Autodesk Fusion 360 part; units mm, degrees
(part 6 of 40)
  line L2344 (251.8229, 91.113) -> (251.9751, 91.0416) construction
  line L2345 (251.9751, 91.0416) -> (252.0973, 90.9849) construction
  line L2346 (252.0973, 90.9849) -> (252.1892, 90.9427) construction
  line L2347 (252.1892, 90.9427) -> (252.2505, 90.9147) construction
  line L2348 (252.2505, 90.9147) -> (252.2812, 90.9007) construction
  spline S31 degree 5 poles (243.2435, 97.4897) (243.2592, 97.4632) (243.2914, 97.4105) (243.3417, 97.3328) (243.4127, 97.2319) (243.5068, 97.1094) (243.6047, 96.9894) (243.7049, 96.8711) (243.8064, 96.7536) (243.9087, 96.6366) (244.012, 96.5203) (244.1164, 96.4049) (244.2223, 96.2906) (244.3301, 96.1776) (244.4397, 96.066) (244.551, 95.9556) (244.6636, 95.8463) (244.7775, 95.7378) (244.8923, 95.6302) (245.008, 95.5233) (245.1247, 95.4172) (245.2425, 95.3119) (245.3612, 95.2074) (245.4811, 95.1039) (245.602, 95.0012) (245.7239, 94.8993) (245.8468, 94.7983) (245.9706, 94.698) (246.0953, 94.5985) (246.2208, 94.4997) (246.3471, 94.4016) (246.4743, 94.3043) (246.6023, 94.2077) (246.7311, 94.1119) (246.8608, 94.0168) (246.9912, 93.9224) (247.1225, 93.8288) (247.2544, 93.7358) (247.3872, 93.6436) (247.5206, 93.552) (247.6548, 93.4612) (247.7897, 93.371) (247.9253, 93.2815) (248.0615, 93.1927) (248.1985, 93.1045) (248.3362, 93.0171) (248.4745, 92.9303) (248.6135, 92.8442) (248.7531, 92.7587) (248.8934, 92.6739) (249.0343, 92.5898) (249.1758, 92.5063) (249.318, 92.4235) (249.4608, 92.3413) (249.6041, 92.2597) (249.7481, 92.1788) (249.8927, 92.0986) (250.0378, 92.019) (250.1835, 91.94) (250.3298, 91.8617) (250.4767, 91.784) (250.6241, 91.7069) (250.7721, 91.6305) (250.9206, 91.5547) (251.0697, 91.4795) (251.2193, 91.405) (251.3694, 91.331) (251.5201, 91.2577) (251.6713, 91.1851) (251.8229, 91.113) (251.9751, 91.0416) (252.0973, 90.9849) (252.1892, 90.9427) (252.2505, 90.9147) (252.2812, 90.9007) knots 0 0 0 0 0 0 0.01428571 0.02857143 0.04285714 0.05714286 0.07142857 0.08571429 0.1 0.11428571 0.12857143 0.14285714 0.15714286 0.17142857 0.18571429 0.2 0.21428571 0.22857143 0.24285714 0.25714286 0.27142857 0.28571429 0.3 0.31428571 0.32857143 0.34285714 0.35714286 0.37142857 0.38571429 0.4 0.41428571 0.42857143 0.44285714 0.45714286 0.47142857 0.48571429 0.5 0.51428571 0.52857143 0.54285714 0.55714286 0.57142857 0.58571429 0.6 0.61428571 0.62857143 0.64285714 0.65714286 0.67142857 0.68571429 0.7 0.71428571 0.72857143 0.74285714 0.75714286 0.77142857 0.78571429 0.8 0.81428571 0.82857143 0.84285714 0.85714286 0.87142857 0.88571429 0.9 0.91428571 0.92857143 0.94285714 0.95714286 0.97142857 0.98571429 1 1 1 1 1 1
  line L2349 (243.2435, 97.4897) -> (243.2592, 97.4632) construction
  line L2350 (243.2592, 97.4632) -> (243.2914, 97.4105) construction
  line L2351 (243.2914, 97.4105) -> (243.3417, 97.3328) construction
  line L2352 (243.3417, 97.3328) -> (243.4127, 97.2319) construction
  line L2353 (243.4127, 97.2319) -> (243.5068, 97.1094) construction
  line L2354 (243.5068, 97.1094) -> (243.6047, 96.9894) construction
  line L2355 (243.6047, 96.9894) -> (243.7049, 96.8711) construction
  line L2356 (243.7049, 96.8711) -> (243.8064, 96.7536) construction
  line L2357 (243.8064, 96.7536) -> (243.9087, 96.6366) construction
  line L2358 (243.9087, 96.6366) -> (244.012, 96.5203) construction
  line L2359 (244.012, 96.5203) -> (244.1164, 96.4049) construction
  line L2360 (244.1164, 96.4049) -> (244.2223, 96.2906) construction
  line L2361 (244.2223, 96.2906) -> (244.3301, 96.1776) construction
  line L2362 (244.3301, 96.1776) -> (244.4397, 96.066) construction
  line L2363 (244.4397, 96.066) -> (244.551, 95.9556) construction
  line L2364 (244.551, 95.9556) -> (244.6636, 95.8463) construction
  line L2365 (244.6636, 95.8463) -> (244.7775, 95.7378) construction
  line L2366 (244.7775, 95.7378) -> (244.8923, 95.6302) construction
  line L2367 (244.8923, 95.6302) -> (245.008, 95.5233) construction
  line L2368 (245.008, 95.5233) -> (245.1247, 95.4172) construction
  line L2369 (245.1247, 95.4172) -> (245.2425, 95.3119) construction
  line L2370 (245.2425, 95.3119) -> (245.3612, 95.2074) construction
  line L2371 (245.3612, 95.2074) -> (245.4811, 95.1039) construction
  line L2372 (245.4811, 95.1039) -> (245.602, 95.0012) construction
  line L2373 (245.602, 95.0012) -> (245.7239, 94.8993) construction
  line L2374 (245.7239, 94.8993) -> (245.8468, 94.7983) construction
  line L2375 (245.8468, 94.7983) -> (245.9706, 94.698) construction
  line L2376 (245.9706, 94.698) -> (246.0953, 94.5985) construction
  line L2377 (246.0953, 94.5985) -> (246.2208, 94.4997) construction
  line L2378 (246.2208, 94.4997) -> (246.3471, 94.4016) construction
  line L2379 (246.3471, 94.4016) -> (246.4743, 94.3043) construction
  line L2380 (246.4743, 94.3043) -> (246.6023, 94.2077) construction
  line L2381 (246.6023, 94.2077) -> (246.7311, 94.1119) construction
  line L2382 (246.7311, 94.1119) -> (246.8608, 94.0168) construction
  line L2383 (246.8608, 94.0168) -> (246.9912, 93.9224) construction
  line L2384 (246.9912, 93.9224) -> (247.1225, 93.8288) construction
  line L2385 (247.1225, 93.8288) -> (247.2544, 93.7358) construction
  line L2386 (247.2544, 93.7358) -> (247.3872, 93.6436) construction
  line L2387 (247.3872, 93.6436) -> (247.5206, 93.552) construction
  line L2388 (247.5206, 93.552) -> (247.6548, 93.4612) construction
  line L2389 (247.6548, 93.4612) -> (247.7897, 93.371) construction
  line L2390 (247.7897, 93.371) -> (247.9253, 93.2815) construction
  line L2391 (247.9253, 93.2815) -> (248.0615, 93.1927) construction
  line L2392 (248.0615, 93.1927) -> (248.1985, 93.1045) construction
  line L2393 (248.1985, 93.1045) -> (248.3362, 93.0171) construction
  line L2394 (248.3362, 93.0171) -> (248.4745, 92.9303) construction
  line L2395 (248.4745, 92.9303) -> (248.6135, 92.8442) construction
  line L2396 (248.6135, 92.8442) -> (248.7531, 92.7587) construction
  line L2397 (248.7531, 92.7587) -> (248.8934, 92.6739) construction
  line L2398 (248.8934, 92.6739) -> (249.0343, 92.5898) construction
  line L2399 (249.0343, 92.5898) -> (249.1758, 92.5063) construction
  line L2400 (249.1758, 92.5063) -> (249.318, 92.4235) construction
  line L2401 (249.318, 92.4235) -> (249.4608, 92.3413) construction
  line L2402 (249.4608, 92.3413) -> (249.6041, 92.2597) construction
  line L2403 (249.6041, 92.2597) -> (249.7481, 92.1788) construction
  line L2404 (249.7481, 92.1788) -> (249.8927, 92.0986) construction
  line L2405 (249.8927, 92.0986) -> (250.0378, 92.019) construction
  line L2406 (250.0378, 92.019) -> (250.1835, 91.94) construction
  line L2407 (250.1835, 91.94) -> (250.3298, 91.8617) construction
  line L2408 (250.3298, 91.8617) -> (250.4767, 91.784) construction
  line L2409 (250.4767, 91.784) -> (250.6241, 91.7069) construction
  line L2410 (250.6241, 91.7069) -> (250.7721, 91.6305) construction
  line L2411 (250.7721, 91.6305) -> (250.9206, 91.5547) construction
  line L2412 (250.9206, 91.5547) -> (251.0697, 91.4795) construction
  line L2413 (251.0697, 91.4795) -> (251.2193, 91.405) construction
  line L2414 (251.2193, 91.405) -> (251.3694, 91.331) construction
  line L2415 (251.3694, 91.331) -> (251.5201, 91.2577) construction
  line L2416 (251.5201, 91.2577) -> (251.6713, 91.1851) construction
  line L2417 (251.6713, 91.1851) -> (251.8229, 91.113) construction
  line L2418 (251.8229, 91.113) -> (251.9751, 91.0416) construction
  line L2419 (251.9751, 91.0416) -> (252.0973, 90.9849) construction
  line L2420 (252.0973, 90.9849) -> (252.1892, 90.9427) construction
  line L2421 (252.1892, 90.9427) -> (252.2505, 90.9147) construction
  line L2422 (252.2505, 90.9147) -> (252.2812, 90.9007) construction
  arc A81 (280.7456, 169.9215) -> (279.3511, 174.2132) centre (212.132, 150) ccw
  arc A82 (280.7456, 169.9215) -> (279.3511, 174.2132) centre (212.132, 150) ccw
  spline S32 degree 5 poles (268.1665, 174.1948) (268.1948, 174.2071) (268.2518, 174.2308) (268.3382, 174.264) (268.4549, 174.3039) (268.6031, 174.3478) (268.7528, 174.3873) (268.9034, 174.4241) (269.0546, 174.4595) (269.2061, 174.494) (269.358, 174.5274) (269.5103, 174.5594) (269.6632, 174.5896) (269.8168, 174.6176) (269.9711, 174.6435) (270.126, 174.6674) (270.2814, 174.6897) (270.4372, 174.7105) (270.5934, 174.7301) (270.7499, 174.7485) (270.9067, 174.7658) (271.0638, 174.7818) (271.2213, 174.7965) (271.3791, 174.8098) (271.5373, 174.8218) (271.6958, 174.8325) (271.8546, 174.842) (272.0137, 174.8504) (272.1731, 174.8577) (272.3327, 174.8638) (272.4925, 174.8689) (272.6526, 174.8729) (272.8129, 174.8757) (272.9735, 174.8776) (273.1343, 174.8783) (273.2953, 174.878) (273.4565, 174.8766) (273.6179, 174.8742) (273.7795, 174.8708) (273.9413, 174.8665) (274.1032, 174.8611) (274.2654, 174.8548) (274.4277, 174.8475) (274.5901, 174.8392) (274.7527, 174.83) (274.9155, 174.8199) (275.0784, 174.8088) (275.2415, 174.7967) (275.4047, 174.7838) (275.568, 174.77) (275.7315, 174.7552) (275.8951, 174.7396) (276.0588, 174.723) (276.2226, 174.7056) (276.3865, 174.6873) (276.5505, 174.6681) (276.7146, 174.648) (276.8788, 174.6271) (277.0431, 174.6054) (277.2075, 174.5828) (277.372, 174.5593) (277.5366, 174.535) (277.7012, 174.5098) (277.866, 174.4839) (278.0307, 174.4571) (278.1956, 174.4294) (278.3605, 174.401) (278.5255, 174.3718) (278.6905, 174.3417) (278.8556, 174.3108) (279.0207, 174.2792) (279.1528, 174.2532) (279.2519, 174.2334) (279.318, 174.22) (279.3511, 174.2132) knots 0 0 0 0 0 0 0.01428571 0.02857143 0.04285714 0.05714286 0.07142857 0.08571429 0.1 0.11428571 0.12857143 0.14285714 0.15714286 0.17142857 0.18571429 0.2 0.21428571 0.22857143 0.24285714 0.25714286 0.27142857 0.28571429 0.3 0.31428571 0.32857143 0.34285714 0.35714286 0.37142857 0.38571429 0.4 0.41428571 0.42857143 0.44285714 0.45714286 0.47142857 0.48571429 0.5 0.51428571 0.52857143 0.54285714 0.55714286 0.57142857 0.58571429 0.6 0.61428571 0.62857143 0.64285714 0.65714286 0.67142857 0.68571429 0.7 0.71428571 0.72857143 0.74285714 0.75714286 0.77142857 0.78571429 0.8 0.81428571 0.82857143 0.84285714 0.85714286 0.87142857 0.88571429 0.9 0.91428571 0.92857143 0.94285714 0.95714286 0.97142857 0.98571429 1 1 1 1 1 1
  line L2423 (268.1665, 174.1948) -> (268.1948, 174.2071) construction
  line L2424 (268.1948, 174.2071) -> (268.2518, 174.2308) construction
  line L2425 (268.2518, 174.2308) -> (268.3382, 174.264) construction
  line L2426 (268.3382, 174.264) -> (268.4549, 174.3039) construction
  line L2427 (268.4549, 174.3039) -> (268.6031, 174.3478) construction
  line L2428 (268.6031, 174.3478) -> (268.7528, 174.3873) construction
  line L2429 (268.7528, 174.3873) -> (268.9034, 174.4241) construction
  line L2430 (268.9034, 174.4241) -> (269.0546, 174.4595) construction
  line L2431 (269.0546, 174.4595) -> (269.2061, 174.494) construction
  line L2432 (269.2061, 174.494) -> (269.358, 174.5274) construction
  line L2433 (269.358, 174.5274) -> (269.5103, 174.5594) construction
  line L2434 (269.5103, 174.5594) -> (269.6632, 174.5896) construction
  line L2435 (269.6632, 174.5896) -> (269.8168, 174.6176) construction
  line L2436 (269.8168, 174.6176) -> (269.9711, 174.6435) construction
  line L2437 (269.9711, 174.6435) -> (270.126, 174.6674) construction
  line L2438 (270.126, 174.6674) -> (270.2814, 174.6897) construction
  line L2439 (270.2814, 174.6897) -> (270.4372, 174.7105) construction
  line L2440 (270.4372, 174.7105) -> (270.5934, 174.7301) construction
  line L2441 (270.5934, 174.7301) -> (270.7499, 174.7485) construction
  line L2442 (270.7499, 174.7485) -> (270.9067, 174.7658) construction
  line L2443 (270.9067, 174.7658) -> (271.0638, 174.7818) construction
  line L2444 (271.0638, 174.7818) -> (271.2213, 174.7965) construction
  line L2445 (271.2213, 174.7965) -> (271.3791, 174.8098) construction
  line L2446 (271.3791, 174.8098) -> (271.5373, 174.8218) construction
  line L2447 (271.5373, 174.8218) -> (271.6958, 174.8325) construction
  line L2448 (271.6958, 174.8325) -> (271.8546, 174.842) construction
  line L2449 (271.8546, 174.842) -> (272.0137, 174.8504) construction
  line L2450 (272.0137, 174.8504) -> (272.1731, 174.8577) construction
  line L2451 (272.1731, 174.8577) -> (272.3327, 174.8638) construction
  line L2452 (272.3327, 174.8638) -> (272.4925, 174.8689) construction
  line L2453 (272.4925, 174.8689) -> (272.6526, 174.8729) construction
  line L2454 (272.6526, 174.8729) -> (272.8129, 174.8757) construction
  line L2455 (272.8129, 174.8757) -> (272.9735, 174.8776) construction
  line L2456 (272.9735, 174.8776) -> (273.1343, 174.8783) construction
  line L2457 (273.1343, 174.8783) -> (273.2953, 174.878) construction
  line L2458 (273.2953, 174.878) -> (273.4565, 174.8766) construction
  line L2459 (273.4565, 174.8766) -> (273.6179, 174.8742) construction
  line L2460 (273.6179, 174.8742) -> (273.7795, 174.8708) construction
  line L2461 (273.7795, 174.8708) -> (273.9413, 174.8665) construction
  line L2462 (273.9413, 174.8665) -> (274.1032, 174.8611) construction
  line L2463 (274.1032, 174.8611) -> (274.2654, 174.8548) construction
  line L2464 (274.2654, 174.8548) -> (274.4277, 174.8475) construction
  line L2465 (274.4277, 174.8475) -> (274.5901, 174.8392) construction
  line L2466 (274.5901, 174.8392) -> (274.7527, 174.83) construction
  line L2467 (274.7527, 174.83) -> (274.9155, 174.8199) construction
  line L2468 (274.9155, 174.8199) -> (275.0784, 174.8088) construction
  line L2469 (275.0784, 174.8088) -> (275.2415, 174.7967) construction
  line L2470 (275.2415, 174.7967) -> (275.4047, 174.7838) construction
  line L2471 (275.4047, 174.7838) -> (275.568, 174.77) construction
  line L2472 (275.568, 174.77) -> (275.7315, 174.7552) construction
  line L2473 (275.7315, 174.7552) -> (275.8951, 174.7396) construction
  line L2474 (275.8951, 174.7396) -> (276.0588, 174.723) construction
  line L2475 (276.0588, 174.723) -> (276.2226, 174.7056) construction
  line L2476 (276.2226, 174.7056) -> (276.3865, 174.6873) construction
  line L2477 (276.3865, 174.6873) -> (276.5505, 174.6681) construction
  line L2478 (276.5505, 174.6681) -> (276.7146, 174.648) construction
  line L2479 (276.7146, 174.648) -> (276.8788, 174.6271) construction
  line L2480 (276.8788, 174.6271) -> (277.0431, 174.6054) construction
  line L2481 (277.0431, 174.6054) -> (277.2075, 174.5828) construction
  line L2482 (277.2075, 174.5828) -> (277.372, 174.5593) construction
  line L2483 (277.372, 174.5593) -> (277.5366, 174.535) construction
  line L2484 (277.5366, 174.535) -> (277.7012, 174.5098) construction
  line L2485 (277.7012, 174.5098) -> (277.866, 174.4839) construction
  line L2486 (277.866, 174.4839) -> (278.0307, 174.4571) construction
  line L2487 (278.0307, 174.4571) -> (278.1956, 174.4294) construction
  line L2488 (278.1956, 174.4294) -> (278.3605, 174.401) construction
  line L2489 (278.3605, 174.401) -> (278.5255, 174.3718) construction
  line L2490 (278.5255, 174.3718) -> (278.6905, 174.3417) construction
  line L2491 (278.6905, 174.3417) -> (278.8556, 174.3108) construction
  line L2492 (278.8556, 174.3108) -> (279.0207, 174.2792) construction
  line L2493 (279.0207, 174.2792) -> (279.1528, 174.2532) construction
  line L2494 (279.1528, 174.2532) -> (279.2519, 174.2334) construction
  line L2495 (279.2519, 174.2334) -> (279.318, 174.22) construction
  line L2496 (279.318, 174.22) -> (279.3511, 174.2132) construction
  spline S33 degree 5 poles (268.1665, 174.1948) (268.1948, 174.2071) (268.2518, 174.2308) (268.3382, 174.264) (268.4549, 174.3039) (268.6031, 174.3478) (268.7528, 174.3873) (268.9034, 174.4241) (269.0546, 174.4595) (269.2061, 174.494) (269.358, 174.5274) (269.5103, 174.5594) (269.6632, 174.5896) (269.8168, 174.6176) (269.9711, 174.6435) (270.126, 174.6674) (270.2814, 174.6897) (270.4372, 174.7105) (270.5934, 174.7301) (270.7499, 174.7485) (270.9067, 174.7658) (271.0638, 174.7818) (271.2213, 174.7965) (271.3791, 174.8098) (271.5373, 174.8218) (271.6958, 174.8325) (271.8546, 174.842) (272.0137, 174.8504) (272.1731, 174.8577) (272.3327, 174.8638) (272.4925, 174.8689) (272.6526, 174.8729) (272.8129, 174.8757) (272.9735, 174.8776) (273.1343, 174.8783) (273.2953, 174.878) (273.4565, 174.8766) (273.6179, 174.8742) (273.7795, 174.8708) (273.9413, 174.8665) (274.1032, 174.8611) (274.2654, 174.8548) (274.4277, 174.8475) (274.5901, 174.8392) (274.7527, 174.83) (274.9155, 174.8199) (275.0784, 174.8088) (275.2415, 174.7967) (275.4047, 174.7838) (275.568, 174.77) (275.7315, 174.7552) (275.8951, 174.7396) (276.0588, 174.723) (276.2226, 174.7056) (276.3865, 174.6873) (276.5505, 174.6681) (276.7146, 174.648) (276.8788, 174.6271) (277.0431, 174.6054) (277.2075, 174.5828) (277.372, 174.5593) (277.5366, 174.535) (277.7012, 174.5098) (277.866, 174.4839) (278.0307, 174.4571) (278.1956, 174.4294) (278.3605, 174.401) (278.5255, 174.3718) (278.6905, 174.3417) (278.8556, 174.3108) (279.0207, 174.2792) (279.1528, 174.2532) (279.2519, 174.2334) (279.318, 174.22) (279.3511, 174.2132) knots 0 0 0 0 0 0 0.01428571 0.02857143 0.04285714 0.05714286 0.07142857 0.08571429 0.1 0.11428571 0.12857143 0.14285714 0.15714286 0.17142857 0.18571429 0.2 0.21428571 0.22857143 0.24285714 0.25714286 0.27142857 0.28571429 0.3 0.31428571 0.32857143 0.34285714 0.35714286 0.37142857 0.38571429 0.4 0.41428571 0.42857143 0.44285714 0.45714286 0.47142857 0.48571429 0.5 0.51428571 0.52857143 0.54285714 0.55714286 0.57142857 0.58571429 0.6 0.61428571 0.62857143 0.64285714 0.65714286 0.67142857 0.68571429 0.7 0.71428571 0.72857143 0.74285714 0.75714286 0.77142857 0.78571429 0.8 0.81428571 0.82857143 0.84285714 0.85714286 0.87142857 0.88571429 0.9 0.91428571 0.92857143 0.94285714 0.95714286 0.97142857 0.98571429 1 1 1 1 1 1
  line L2497 (268.1665, 174.1948) -> (268.1948, 174.2071) construction
  line L2498 (268.1948, 174.2071) -> (268.2518, 174.2308) construction
  line L2499 (268.2518, 174.2308) -> (268.3382, 174.264) construction
  line L2500 (268.3382, 174.264) -> (268.4549, 174.3039) construction
  line L2501 (268.4549, 174.3039) -> (268.6031, 174.3478) construction
  line L2502 (268.6031, 174.3478) -> (268.7528, 174.3873) construction
  line L2503 (268.7528, 174.3873) -> (268.9034, 174.4241) construction
  line L2504 (268.9034, 174.4241) -> (269.0546, 174.4595) construction
  line L2505 (269.0546, 174.4595) -> (269.2061, 174.494) construction
  line L2506 (269.2061, 174.494) -> (269.358, 174.5274) construction
  line L2507 (269.358, 174.5274) -> (269.5103, 174.5594) construction
  line L2508 (269.5103, 174.5594) -> (269.6632, 174.5896) construction
  line L2509 (269.6632, 174.5896) -> (269.8168, 174.6176) construction
  line L2510 (269.8168, 174.6176) -> (269.9711, 174.6435) construction
  line L2511 (269.9711, 174.6435) -> (270.126, 174.6674) construction
  line L2512 (270.126, 174.6674) -> (270.2814, 174.6897) construction
  line L2513 (270.2814, 174.6897) -> (270.4372, 174.7105) construction
  line L2514 (270.4372, 174.7105) -> (270.5934, 174.7301) construction
  line L2515 (270.5934, 174.7301) -> (270.7499, 174.7485) construction
  line L2516 (270.7499, 174.7485) -> (270.9067, 174.7658) construction
  line L2517 (270.9067, 174.7658) -> (271.0638, 174.7818) construction
  line L2518 (271.0638, 174.7818) -> (271.2213, 174.7965) construction
  line L2519 (271.2213, 174.7965) -> (271.3791, 174.8098) construction
  line L2520 (271.3791, 174.8098) -> (271.5373, 174.8218) construction
  line L2521 (271.5373, 174.8218) -> (271.6958, 174.8325) construction
  line L2522 (271.6958, 174.8325) -> (271.8546, 174.842) construction
  line L2523 (271.8546, 174.842) -> (272.0137, 174.8504) construction
  line L2524 (272.0137, 174.8504) -> (272.1731, 174.8577) construction
  line L2525 (272.1731, 174.8577) -> (272.3327, 174.8638) construction
  line L2526 (272.3327, 174.8638) -> (272.4925, 174.8689) construction
  line L2527 (272.4925, 174.8689) -> (272.6526, 174.8729) construction
  line L2528 (272.6526, 174.8729) -> (272.8129, 174.8757) construction
  line L2529 (272.8129, 174.8757) -> (272.9735, 174.8776) construction
  line L2530 (272.9735, 174.8776) -> (273.1343, 174.8783) construction
  line L2531 (273.1343, 174.8783) -> (273.2953, 174.878) construction
  line L2532 (273.2953, 174.878) -> (273.4565, 174.8766) construction
  line L2533 (273.4565, 174.8766) -> (273.6179, 174.8742) construction
  line L2534 (273.6179, 174.8742) -> (273.7795, 174.8708) construction
  line L2535 (273.7795, 174.8708) -> (273.9413, 174.8665) construction
  line L2536 (273.9413, 174.8665) -> (274.1032, 174.8611) construction
  line L2537 (274.1032, 174.8611) -> (274.2654, 174.8548) construction
  line L2538 (274.2654, 174.8548) -> (274.4277, 174.8475) construction
  line L2539 (274.4277, 174.8475) -> (274.5901, 174.8392) construction
  line L2540 (274.5901, 174.8392) -> (274.7527, 174.83) construction
  line L2541 (274.7527, 174.83) -> (274.9155, 174.8199) construction
  line L2542 (274.9155, 174.8199) -> (275.0784, 174.8088) construction
  line L2543 (275.0784, 174.8088) -> (275.2415, 174.7967) construction
  line L2544 (275.2415, 174.7967) -> (275.4047, 174.7838) construction
  line L2545 (275.4047, 174.7838) -> (275.568, 174.77) construction
  line L2546 (275.568, 174.77) -> (275.7315, 174.7552) construction
  line L2547 (275.7315, 174.7552) -> (275.8951, 174.7396) construction
  line L2548 (275.8951, 174.7396) -> (276.0588, 174.723) construction
  line L2549 (276.0588, 174.723) -> (276.2226, 174.7056) construction
  line L2550 (276.2226, 174.7056) -> (276.3865, 174.6873) construction
  line L2551 (276.3865, 174.6873) -> (276.5505, 174.6681) construction
  line L2552 (276.5505, 174.6681) -> (276.7146, 174.648) construction
  line L2553 (276.7146, 174.648) -> (276.8788, 174.6271) construction
  line L2554 (276.8788, 174.6271) -> (277.0431, 174.6054) construction
  line L2555 (277.0431, 174.6054) -> (277.2075, 174.5828) construction
  line L2556 (277.2075, 174.5828) -> (277.372, 174.5593) construction
  line L2557 (277.372, 174.5593) -> (277.5366, 174.535) construction
  line L2558 (277.5366, 174.535) -> (277.7012, 174.5098) construction
  line L2559 (277.7012, 174.5098) -> (277.866, 174.4839) construction
  line L2560 (277.866, 174.4839) -> (278.0307, 174.4571) construction
  line L2561 (278.0307, 174.4571) -> (278.1956, 174.4294) construction
  line L2562 (278.1956, 174.4294) -> (278.3605, 174.401) construction
  line L2563 (278.3605, 174.401) -> (278.5255, 174.3718) construction
  line L2564 (278.5255, 174.3718) -> (278.6905, 174.3417) construction
  line L2565 (278.6905, 174.3417) -> (278.8556, 174.3108) construction
  line L2566 (278.8556, 174.3108) -> (279.0207, 174.2792) construction
  line L2567 (279.0207, 174.2792) -> (279.1528, 174.2532) construction
  line L2568 (279.1528, 174.2532) -> (279.2519, 174.2334) construction
  line L2569 (279.2519, 174.2334) -> (279.318, 174.22) construction
  line L2570 (279.318, 174.22) -> (279.3511, 174.2132) construction
  line L2571 (270.0943, 163.005) -> (271.6862, 163.3622)
  line L2572 (270.0943, 163.005) -> (271.6862, 163.3622)
  arc A83 (270.0943, 163.005) -> (268.567, 160.6816) centre (270.5321, 161.0535) ccw
  arc A84 (268.5789, 106.2) -> (271.2313, 109.8508) centre (212.132, 150) ccw
  arc A85 (268.5789, 106.2) -> (271.2313, 109.8508) centre (212.132, 150) ccw
  arc A86 (270.0943, 163.005) -> (268.567, 160.6816) centre (270.5321, 161.0535) ccw
  line L2573 (225.137, 207.9623) -> (225.4942, 209.5542)
  arc A87 (201.4504, 93.565) -> (204.8514, 93.0263) centre (212.132, 150) ccw
  arc A88 (201.4504, 93.565) -> (204.8514, 93.0263) centre (212.132, 150) ccw
  arc A89 (206.5892, 90.8558) -> (204.8514, 93.0263) centre (204.5979, 91.0425) ccw
  arc A90 (206.5892, 90.8558) -> (204.8514, 93.0263) centre (204.5979, 91.0425) ccw
  arc A91 (187.6019, 201.9354) -> (188.5839, 204.5366) centre (186.7478, 203.7438) ccw
  line L2574 (188.5839, 204.5366) -> (187.9372, 206.0345)
  line L2575 (225.137, 207.9623) -> (225.4942, 209.5542)
  arc A92 (222.8136, 206.435) -> (225.137, 207.9623) centre (223.1855, 208.4001) ccw
  arc A93 (222.8136, 206.435) -> (225.137, 207.9623) centre (223.1855, 208.4001) ccw
  arc A94 (222.8136, 206.435) -> (219.4126, 206.9737) centre (212.132, 150) ccw
  arc A95 (222.8136, 206.435) -> (219.4126, 206.9737) centre (212.132, 150) ccw
  spline S34 degree 5 poles (225.4942, 209.5542) (225.501, 209.5843) (225.5153, 209.6444) (225.5391, 209.7338) (225.5755, 209.8517) (225.6271, 209.9973) (225.6831, 210.1416) (225.7419, 210.2852) (225.8021, 210.4283) (225.8633, 210.5711) (225.9255, 210.7136) (225.9891, 210.8557) (226.0546, 210.9971) (226.1222, 211.1379) (226.192, 211.2779) (226.2636, 211.4173) (226.337, 211.5561) (226.4117, 211.6944) (226.4877, 211.8322) (226.5647, 211.9697) (226.6429, 212.1067) (226.7224, 212.2432) (226.8031, 212.3792) (226.885, 212.5148) (226.9683, 212.6498) (227.0528, 212.7843) (227.1384, 212.9184) (227.2252, 213.052) (227.313, 213.1852) (227.4018, 213.318) (227.4917, 213.4503) (227.5826, 213.5821) (227.6745, 213.7135) (227.7674, 213.8445) (227.8613, 213.975) (227.9562, 214.105) (228.052, 214.2346) (228.1488, 214.3638) (228.2466, 214.4926) (228.3452, 214.6209) (228.4447, 214.7488) (228.5451, 214.8762) (228.6464, 215.0032) (228.7486, 215.1298) (228.8516, 215.256) (228.9555, 215.3817) (229.0603, 215.507) (229.1658, 215.6318) (229.2722, 215.7562) (229.3794, 215.8802) (229.4875, 216.0038) (229.5963, 216.1269) (229.7059, 216.2497) (229.8162, 216.3719) (229.9274, 216.4938) (230.0393, 216.6152) (230.152, 216.7362) (230.2655, 216.8568) (230.3797, 216.9769) (230.4946, 217.0966) (230.6102, 217.2159) (230.7266, 217.3347) (230.8438, 217.4531) (230.9616, 217.5711) (231.0801, 217.6887) (231.1994, 217.8058) (231.3193, 217.9225) (231.4399, 218.0388) (231.5613, 218.1546) (231.6832, 218.27) (231.8059, 218.385) (231.9046, 218.4767) (231.9789, 218.5452) (232.0286, 218.5908) (232.0535, 218.6136) knots 0 0 0 0 0 0 0.01428571 0.02857143 0.04285714 0.05714286 0.07142857 0.08571429 0.1 0.11428571 0.12857143 0.14285714 0.15714286 0.17142857 0.18571429 0.2 0.21428571 0.22857143 0.24285714 0.25714286 0.27142857 0.28571429 0.3 0.31428571 0.32857143 0.34285714 0.35714286 0.37142857 0.38571429 0.4 0.41428571 0.42857143 0.44285714 0.45714286 0.47142857 0.48571429 0.5 0.51428571 0.52857143 0.54285714 0.55714286 0.57142857 0.58571429 0.6 0.61428571 0.62857143 0.64285714 0.65714286 0.67142857 0.68571429 0.7 0.71428571 0.72857143 0.74285714 0.75714286 0.77142857 0.78571429 0.8 0.81428571 0.82857143 0.84285714 0.85714286 0.87142857 0.88571429 0.9 0.91428571 0.92857143 0.94285714 0.95714286 0.97142857 0.98571429 1 1 1 1 1 1
  line L2576 (225.4942, 209.5542) -> (225.501, 209.5843) construction
  line L2577 (225.501, 209.5843) -> (225.5153, 209.6444) construction
  line L2578 (225.5153, 209.6444) -> (225.5391, 209.7338) construction
  line L2579 (225.5391, 209.7338) -> (225.5755, 209.8517) construction
  line L2580 (225.5755, 209.8517) -> (225.6271, 209.9973) construction
  line L2581 (225.6271, 209.9973) -> (225.6831, 210.1416) construction
  line L2582 (225.6831, 210.1416) -> (225.7419, 210.2852) construction
  line L2583 (225.7419, 210.2852) -> (225.8021, 210.4283) construction
  line L2584 (225.8021, 210.4283) -> (225.8633, 210.5711) construction
  line L2585 (225.8633, 210.5711) -> (225.9255, 210.7136) construction
  line L2586 (225.9255, 210.7136) -> (225.9891, 210.8557) construction
  line L2587 (225.9891, 210.8557) -> (226.0546, 210.9971) construction
  line L2588 (226.0546, 210.9971) -> (226.1222, 211.1379) construction
  line L2589 (226.1222, 211.1379) -> (226.192, 211.2779) construction
  line L2590 (226.192, 211.2779) -> (226.2636, 211.4173) construction
  line L2591 (226.2636, 211.4173) -> (226.337, 211.5561) construction
  line L2592 (226.337, 211.5561) -> (226.4117, 211.6944) construction
  line L2593 (226.4117, 211.6944) -> (226.4877, 211.8322) construction
  line L2594 (226.4877, 211.8322) -> (226.5647, 211.9697) construction
  line L2595 (226.5647, 211.9697) -> (226.6429, 212.1067) construction
  line L2596 (226.6429, 212.1067) -> (226.7224, 212.2432) construction
  line L2597 (226.7224, 212.2432) -> (226.8031, 212.3792) construction
  line L2598 (226.8031, 212.3792) -> (226.885, 212.5148) construction
  line L2599 (226.885, 212.5148) -> (226.9683, 212.6498) construction
  line L2600 (226.9683, 212.6498) -> (227.0528, 212.7843) construction
  line L2601 (227.0528, 212.7843) -> (227.1384, 212.9184) construction
  line L2602 (227.1384, 212.9184) -> (227.2252, 213.052) construction
  line L2603 (227.2252, 213.052) -> (227.313, 213.1852) construction
  line L2604 (227.313, 213.1852) -> (227.4018, 213.318) construction
  line L2605 (227.4018, 213.318) -> (227.4917, 213.4503) construction
  line L2606 (227.4917, 213.4503) -> (227.5826, 213.5821) construction
  line L2607 (227.5826, 213.5821) -> (227.6745, 213.7135) construction
  line L2608 (227.6745, 213.7135) -> (227.7674, 213.8445) construction
  line L2609 (227.7674, 213.8445) -> (227.8613, 213.975) construction
  line L2610 (227.8613, 213.975) -> (227.9562, 214.105) construction
  line L2611 (227.9562, 214.105) -> (228.052, 214.2346) construction
  line L2612 (228.052, 214.2346) -> (228.1488, 214.3638) construction
  line L2613 (228.1488, 214.3638) -> (228.2466, 214.4926) construction
  line L2614 (228.2466, 214.4926) -> (228.3452, 214.6209) construction
  line L2615 (228.3452, 214.6209) -> (228.4447, 214.7488) construction
  line L2616 (228.4447, 214.7488) -> (228.5451, 214.8762) construction
  line L2617 (228.5451, 214.8762) -> (228.6464, 215.0032) construction
  line L2618 (228.6464, 215.0032) -> (228.7486, 215.1298) construction
  line L2619 (228.7486, 215.1298) -> (228.8516, 215.256) construction
  line L2620 (228.8516, 215.256) -> (228.9555, 215.3817) construction
  line L2621 (228.9555, 215.3817) -> (229.0603, 215.507) construction
  line L2622 (229.0603, 215.507) -> (229.1658, 215.6318) construction
  line L2623 (229.1658, 215.6318) -> (229.2722, 215.7562) construction
  line L2624 (229.2722, 215.7562) -> (229.3794, 215.8802) construction
  line L2625 (229.3794, 215.8802) -> (229.4875, 216.0038) construction
  line L2626 (229.4875, 216.0038) -> (229.5963, 216.1269) construction
  line L2627 (229.5963, 216.1269) -> (229.7059, 216.2497) construction
  line L2628 (229.7059, 216.2497) -> (229.8162, 216.3719) construction
  line L2629 (229.8162, 216.3719) -> (229.9274, 216.4938) construction
  line L2630 (229.9274, 216.4938) -> (230.0393, 216.6152) construction
  line L2631 (230.0393, 216.6152) -> (230.152, 216.7362) construction
  line L2632 (230.152, 216.7362) -> (230.2655, 216.8568) construction
  line L2633 (230.2655, 216.8568) -> (230.3797, 216.9769) construction
  line L2634 (230.3797, 216.9769) -> (230.4946, 217.0966) construction
  line L2635 (230.4946, 217.0966) -> (230.6102, 217.2159) construction
  line L2636 (230.6102, 217.2159) -> (230.7266, 217.3347) construction
  line L2637 (230.7266, 217.3347) -> (230.8438, 217.4531) construction
  line L2638 (230.8438, 217.4531) -> (230.9616, 217.5711) construction
  line L2639 (230.9616, 217.5711) -> (231.0801, 217.6887) construction
  line L2640 (231.0801, 217.6887) -> (231.1994, 217.8058) construction
  line L2641 (231.1994, 217.8058) -> (231.3193, 217.9225) construction
  line L2642 (231.3193, 217.9225) -> (231.4399, 218.0388) construction
  line L2643 (231.4399, 218.0388) -> (231.5613, 218.1546) construction
  line L2644 (231.5613, 218.1546) -> (231.6832, 218.27) construction
  line L2645 (231.6832, 218.27) -> (231.8059, 218.385) construction
  line L2646 (231.8059, 218.385) -> (231.9046, 218.4767) construction
  line L2647 (231.9046, 218.4767) -> (231.9789, 218.5452) construction
  line L2648 (231.9789, 218.5452) -> (232.0286, 218.5908) construction
  line L2649 (232.0286, 218.5908) -> (232.0535, 218.6136) construction
  arc A96 (187.6019, 201.9354) -> (188.5839, 204.5366) centre (186.7478, 203.7438) ccw
  spline S35 degree 5 poles (225.4942, 209.5542) (225.501, 209.5843) (225.5153, 209.6444) (225.5391, 209.7338) (225.5755, 209.8517) (225.6271, 209.9973) (225.6831, 210.1416) (225.7419, 210.2852) (225.8021, 210.4283) (225.8633, 210.5711) (225.9255, 210.7136) (225.9891, 210.8557) (226.0546, 210.9971) (226.1222, 211.1379) (226.192, 211.2779) (226.2636, 211.4173) (226.337, 211.5561) (226.4117, 211.6944) (226.4877, 211.8322) (226.5647, 211.9697) (226.6429, 212.1067) (226.7224, 212.2432) (226.8031, 212.3792) (226.885, 212.5148) (226.9683, 212.6498) (227.0528, 212.7843) (227.1384, 212.9184) (227.2252, 213.052) (227.313, 213.1852) (227.4018, 213.318) (227.4917, 213.4503) (227.5826, 213.5821) (227.6745, 213.7135) (227.7674, 213.8445) (227.8613, 213.975) (227.9562, 214.105) (228.052, 214.2346) (228.1488, 214.3638) (228.2466, 214.4926) (228.3452, 214.6209) (228.4447, 214.7488) (228.5451, 214.8762) (228.6464, 215.0032) (228.7486, 215.1298) (228.8516, 215.256) (228.9555, 215.3817) (229.0603, 215.507) (229.1658, 215.6318) (229.2722, 215.7562) (229.3794, 215.8802) (229.4875, 216.0038) (229.5963, 216.1269) (229.7059, 216.2497) (229.8162, 216.3719) (229.9274, 216.4938) (230.0393, 216.6152) (230.152, 216.7362) (230.2655, 216.8568) (230.3797, 216.9769) (230.4946, 217.0966) (230.6102, 217.2159) (230.7266, 217.3347) (230.8438, 217.4531) (230.9616, 217.5711) (231.0801, 217.6887) (231.1994, 217.8058) (231.3193, 217.9225) (231.4399, 218.0388) (231.5613, 218.1546) (231.6832, 218.27) (231.8059, 218.385) (231.9046, 218.4767) (231.9789, 218.5452) (232.0286, 218.5908) (232.0535, 218.6136) knots 0 0 0 0 0 0 0.01428571 0.02857143 0.04285714 0.05714286 0.07142857 0.08571429 0.1 0.11428571 0.12857143 0.14285714 0.15714286 0.17142857 0.18571429 0.2 0.21428571 0.22857143 0.24285714 0.25714286 0.27142857 0.28571429 0.3 0.31428571 0.32857143 0.34285714 0.35714286 0.37142857 0.38571429 0.4 0.41428571 0.42857143 0.44285714 0.45714286 0.47142857 0.48571429 0.5 0.51428571 0.52857143 0.54285714 0.55714286 0.57142857 0.58571429 0.6 0.61428571 0.62857143 0.64285714 0.65714286 0.67142857 0.68571429 0.7 0.71428571 0.72857143 0.74285714 0.75714286 0.77142857 0.78571429 0.8 0.81428571 0.82857143 0.84285714 0.85714286 0.87142857 0.88571429 0.9 0.91428571 0.92857143 0.94285714 0.95714286 0.97142857 0.98571429 1 1 1 1 1 1
  line L2650 (225.4942, 209.5542) -> (225.501, 209.5843) construction
  line L2651 (225.501, 209.5843) -> (225.5153, 209.6444) construction
  line L2652 (225.5153, 209.6444) -> (225.5391, 209.7338) construction
  line L2653 (225.5391, 209.7338) -> (225.5755, 209.8517) construction
  line L2654 (225.5755, 209.8517) -> (225.6271, 209.9973) construction
  line L2655 (225.6271, 209.9973) -> (225.6831, 210.1416) construction
  line L2656 (225.6831, 210.1416) -> (225.7419, 210.2852) construction
  line L2657 (225.7419, 210.2852) -> (225.8021, 210.4283) construction
  line L2658 (225.8021, 210.4283) -> (225.8633, 210.5711) construction
  line L2659 (225.8633, 210.5711) -> (225.9255, 210.7136) construction
  line L2660 (225.9255, 210.7136) -> (225.9891, 210.8557) construction
  line L2661 (225.9891, 210.8557) -> (226.0546, 210.9971) construction
  line L2662 (226.0546, 210.9971) -> (226.1222, 211.1379) construction
  line L2663 (226.1222, 211.1379) -> (226.192, 211.2779) construction
  line L2664 (226.192, 211.2779) -> (226.2636, 211.4173) construction
  line L2665 (226.2636, 211.4173) -> (226.337, 211.5561) construction
  line L2666 (226.337, 211.5561) -> (226.4117, 211.6944) construction
  line L2667 (226.4117, 211.6944) -> (226.4877, 211.8322) construction
  line L2668 (226.4877, 211.8322) -> (226.5647, 211.9697) construction
  line L2669 (226.5647, 211.9697) -> (226.6429, 212.1067) construction
  line L2670 (226.6429, 212.1067) -> (226.7224, 212.2432) construction
  line L2671 (226.7224, 212.2432) -> (226.8031, 212.3792) construction
  line L2672 (226.8031, 212.3792) -> (226.885, 212.5148) construction
  line L2673 (226.885, 212.5148) -> (226.9683, 212.6498) construction
  line L2674 (226.9683, 212.6498) -> (227.0528, 212.7843) construction
  line L2675 (227.0528, 212.7843) -> (227.1384, 212.9184) construction
  line L2676 (227.1384, 212.9184) -> (227.2252, 213.052) construction
  line L2677 (227.2252, 213.052) -> (227.313, 213.1852) construction
  line L2678 (227.313, 213.1852) -> (227.4018, 213.318) construction
  line L2679 (227.4018, 213.318) -> (227.4917, 213.4503) construction
  line L2680 (227.4917, 213.4503) -> (227.5826, 213.5821) construction
  line L2681 (227.5826, 213.5821) -> (227.6745, 213.7135) construction
  line L2682 (227.6745, 213.7135) -> (227.7674, 213.8445) construction
  line L2683 (227.7674, 213.8445) -> (227.8613, 213.975) construction
  line L2684 (227.8613, 213.975) -> (227.9562, 214.105) construction
  line L2685 (227.9562, 214.105) -> (228.052, 214.2346) construction
  line L2686 (228.052, 214.2346) -> (228.1488, 214.3638) construction
  line L2687 (228.1488, 214.3638) -> (228.2466, 214.4926) construction
  line L2688 (228.2466, 214.4926) -> (228.3452, 214.6209) construction
  line L2689 (228.3452, 214.6209) -> (228.4447, 214.7488) construction
  line L2690 (228.4447, 214.7488) -> (228.5451, 214.8762) construction
  line L2691 (228.5451, 214.8762) -> (228.6464, 215.0032) construction
  line L2692 (228.6464, 215.0032) -> (228.7486, 215.1298) construction
  line L2693 (228.7486, 215.1298) -> (228.8516, 215.256) construction
  line L2694 (228.8516, 215.256) -> (228.9555, 215.3817) construction
  line L2695 (228.9555, 215.3817) -> (229.0603, 215.507) construction
  line L2696 (229.0603, 215.507) -> (229.1658, 215.6318) construction
  line L2697 (229.1658, 215.6318) -> (229.2722, 215.7562) construction
  line L2698 (229.2722, 215.7562) -> (229.3794, 215.8802) construction
  line L2699 (229.3794, 215.8802) -> (229.4875, 216.0038) construction
  line L2700 (229.4875, 216.0038) -> (229.5963, 216.1269) construction
  line L2701 (229.5963, 216.1269) -> (229.7059, 216.2497) construction
  line L2702 (229.7059, 216.2497) -> (229.8162, 216.3719) construction
  line L2703 (229.8162, 216.3719) -> (229.9274, 216.4938) construction
  line L2704 (229.9274, 216.4938) -> (230.0393, 216.6152) construction
  line L2705 (230.0393, 216.6152) -> (230.152, 216.7362) construction
  line L2706 (230.152, 216.7362) -> (230.2655, 216.8568) construction
  line L2707 (230.2655, 216.8568) -> (230.3797, 216.9769) construction
  line L2708 (230.3797, 216.9769) -> (230.4946, 217.0966) construction
  line L2709 (230.4946, 217.0966) -> (230.6102, 217.2159) construction
  line L2710 (230.6102, 217.2159) -> (230.7266, 217.3347) construction
  line L2711 (230.7266, 217.3347) -> (230.8438, 217.4531) construction
  line L2712 (230.8438, 217.4531) -> (230.9616, 217.5711) construction
  line L2713 (230.9616, 217.5711) -> (231.0801, 217.6887) construction
  line L2714 (231.0801, 217.6887) -> (231.1994, 217.8058) construction
  line L2715 (231.1994, 217.8058) -> (231.3193, 217.9225) construction
  line L2716 (231.3193, 217.9225) -> (231.4399, 218.0388) construction
  line L2717 (231.4399, 218.0388) -> (231.5613, 218.1546) construction
  line L2718 (231.5613, 218.1546) -> (231.6832, 218.27) construction
  line L2719 (231.6832, 218.27) -> (231.8059, 218.385) construction
  line L2720 (231.8059, 218.385) -> (231.9046, 218.4767) construction
  line L2721 (231.9046, 218.4767) -> (231.9789, 218.5452) construction
  line L2722 (231.9789, 218.5452) -> (232.0286, 218.5908) construction
  line L2723 (232.0286, 218.5908) -> (232.0535, 218.6136) construction
  line L2724 (188.5839, 204.5366) -> (187.9372, 206.0345)
  spline S36 degree 5 poles (187.9372, 93.9655) (187.9249, 93.9372) (187.9012, 93.8802) (187.868, 93.7938) (187.8281, 93.6771) (187.7842, 93.5289) (187.7447, 93.3792) (187.7079, 93.2286) (187.6725, 93.0774) (187.638, 92.9259) (187.6046, 92.774) (187.5726, 92.6217) (187.5424, 92.4688) (187.5144, 92.3152) (187.4885, 92.1609) (187.4646, 92.006) (187.4423, 91.8506) (187.4215, 91.6948) (187.4019, 91.5386) (187.3835, 91.3821) (187.3662, 91.2253) (187.3502, 91.0682) (187.3355, 90.9107) (187.3222, 90.7529) (187.3102, 90.5947) (187.2995, 90.4362) (187.29, 90.2774) (187.2816, 90.1183) (187.2743, 89.9589) (187.2682, 89.7993) (187.2631, 89.6395) (187.2591, 89.4794) (187.2563, 89.3191) (187.2544, 89.1585) (187.2537, 88.9977) (187.254, 88.8367) (187.2554, 88.6755) (187.2578, 88.5141) (187.2612, 88.3525) (187.2655, 88.1907) (187.2709, 88.0288) (187.2772, 87.8666) (187.2845, 87.7043) (187.2928, 87.5419) (187.302, 87.3793) (187.3121, 87.2165) (187.3232, 87.0536) (187.3353, 86.8905) (187.3482, 86.7273) (187.362, 86.564) (187.3768, 86.4005) (187.3924, 86.2369) (187.409, 86.0732) (187.4264, 85.9094) (187.4447, 85.7455) (187.4639, 85.5815) (187.484, 85.4174) (187.5049, 85.2532) (187.5266, 85.0889) (187.5492, 84.9245) (187.5727, 84.76) (187.597, 84.5954) (187.6222, 84.4308) (187.6481, 84.266) (187.6749, 84.1013) (187.7026, 83.9364) (187.731, 83.7715) (187.7602, 83.6065) (187.7903, 83.4415) (187.8212, 83.2764) (187.8528, 83.1113) (187.8788, 82.9792) (187.8986, 82.8801) (187.912, 82.814) (187.9188, 82.7809) knots 0 0 0 0 0 0 0.01428571 0.02857143 0.04285714 0.05714286 0.07142857 0.08571429 0.1 0.11428571 0.12857143 0.14285714 0.15714286 0.17142857 0.18571429 0.2 0.21428571 0.22857143 0.24285714 0.25714286 0.27142857 0.28571429 0.3 0.31428571 0.32857143 0.34285714 0.35714286 0.37142857 0.38571429 0.4 0.41428571 0.42857143 0.44285714 0.45714286 0.47142857 0.48571429 0.5 0.51428571 0.52857143 0.54285714 0.55714286 0.57142857 0.58571429 0.6 0.61428571 0.62857143 0.64285714 0.65714286 0.67142857 0.68571429 0.7 0.71428571 0.72857143 0.74285714 0.75714286 0.77142857 0.78571429 0.8 0.81428571 0.82857143 0.84285714 0.85714286 0.87142857 0.88571429 0.9 0.91428571 0.92857143 0.94285714 0.95714286 0.97142857 0.98571429 1 1 1 1 1 1
  line L2725 (187.9372, 93.9655) -> (187.9249, 93.9372) construction
  line L2726 (187.9249, 93.9372) -> (187.9012, 93.8802) construction
  line L2727 (187.9012, 93.8802) -> (187.868, 93.7938) construction
  line L2728 (187.868, 93.7938) -> (187.8281, 93.6771) construction
  line L2729 (187.8281, 93.6771) -> (187.7842, 93.5289) construction
  line L2730 (187.7842, 93.5289) -> (187.7447, 93.3792) construction
  line L2731 (187.7447, 93.3792) -> (187.7079, 93.2286) construction
  line L2732 (187.7079, 93.2286) -> (187.6725, 93.0774) construction
  line L2733 (187.6725, 93.0774) -> (187.638, 92.9259) construction
  line L2734 (187.638, 92.9259) -> (187.6046, 92.774) construction
  line L2735 (187.6046, 92.774) -> (187.5726, 92.6217) construction
  line L2736 (187.5726, 92.6217) -> (187.5424, 92.4688) construction
  line L2737 (187.5424, 92.4688) -> (187.5144, 92.3152) construction
  line L2738 (187.5144, 92.3152) -> (187.4885, 92.1609) construction
  line L2739 (187.4885, 92.1609) -> (187.4646, 92.006) construction
  line L2740 (187.4646, 92.006) -> (187.4423, 91.8506) construction
  line L2741 (187.4423, 91.8506) -> (187.4215, 91.6948) construction
  line L2742 (187.4215, 91.6948) -> (187.4019, 91.5386) construction
  line L2743 (187.4019, 91.5386) -> (187.3835, 91.3821) construction
  line L2744 (187.3835, 91.3821) -> (187.3662, 91.2253) construction
  line L2745 (187.3662, 91.2253) -> (187.3502, 91.0682) construction
  line L2746 (187.3502, 91.0682) -> (187.3355, 90.9107) construction
  line L2747 (187.3355, 90.9107) -> (187.3222, 90.7529) construction
  line L2748 (187.3222, 90.7529) -> (187.3102, 90.5947) construction
  line L2749 (187.3102, 90.5947) -> (187.2995, 90.4362) construction
  line L2750 (187.2995, 90.4362) -> (187.29, 90.2774) construction
  line L2751 (187.29, 90.2774) -> (187.2816, 90.1183) construction
  line L2752 (187.2816, 90.1183) -> (187.2743, 89.9589) construction
  line L2753 (187.2743, 89.9589) -> (187.2682, 89.7993) construction
  line L2754 (187.2682, 89.7993) -> (187.2631, 89.6395) construction
  line L2755 (187.2631, 89.6395) -> (187.2591, 89.4794) construction
  line L2756 (187.2591, 89.4794) -> (187.2563, 89.3191) construction
  line L2757 (187.2563, 89.3191) -> (187.2544, 89.1585) construction
  line L2758 (187.2544, 89.1585) -> (187.2537, 88.9977) construction
  line L2759 (187.2537, 88.9977) -> (187.254, 88.8367) construction
  line L2760 (187.254, 88.8367) -> (187.2554, 88.6755) construction
  line L2761 (187.2554, 88.6755) -> (187.2578, 88.5141) construction
  line L2762 (187.2578, 88.5141) -> (187.2612, 88.3525) construction
  line L2763 (187.2612, 88.3525) -> (187.2655, 88.1907) construction
  line L2764 (187.2655, 88.1907) -> (187.2709, 88.0288) construction
  line L2765 (187.2709, 88.0288) -> (187.2772, 87.8666) construction
  line L2766 (187.2772, 87.8666) -> (187.2845, 87.7043) construction
  line L2767 (187.2845, 87.7043) -> (187.2928, 87.5419) construction
  line L2768 (187.2928, 87.5419) -> (187.302, 87.3793) construction
  line L2769 (187.302, 87.3793) -> (187.3121, 87.2165) construction
  line L2770 (187.3121, 87.2165) -> (187.3232, 87.0536) construction
  line L2771 (187.3232, 87.0536) -> (187.3353, 86.8905) construction
  line L2772 (187.3353, 86.8905) -> (187.3482, 86.7273) construction
  line L2773 (187.3482, 86.7273) -> (187.362, 86.564) construction
  line L2774 (187.362, 86.564) -> (187.3768, 86.4005) construction
  line L2775 (187.3768, 86.4005) -> (187.3924, 86.2369) construction
  line L2776 (187.3924, 86.2369) -> (187.409, 86.0732) construction
  line L2777 (187.409, 86.0732) -> (187.4264, 85.9094) construction
  line L2778 (187.4264, 85.9094) -> (187.4447, 85.7455) construction
  line L2779 (187.4447, 85.7455) -> (187.4639, 85.5815) construction
  line L2780 (187.4639, 85.5815) -> (187.484, 85.4174) construction
  line L2781 (187.484, 85.4174) -> (187.5049, 85.2532) construction
  line L2782 (187.5049, 85.2532) -> (187.5266, 85.0889) construction
  line L2783 (187.5266, 85.0889) -> (187.5492, 84.9245) construction
  line L2784 (187.5492, 84.9245) -> (187.5727, 84.76) construction
  line L2785 (187.5727, 84.76) -> (187.597, 84.5954) construction
  line L2786 (187.597, 84.5954) -> (187.6222, 84.4308) construction
  line L2787 (187.6222, 84.4308) -> (187.6481, 84.266) construction
  line L2788 (187.6481, 84.266) -> (187.6749, 84.1013) construction
  line L2789 (187.6749, 84.1013) -> (187.7026, 83.9364) construction
  line L2790 (187.7026, 83.9364) -> (187.731, 83.7715) construction
  line L2791 (187.731, 83.7715) -> (187.7602, 83.6065) construction
  line L2792 (187.7602, 83.6065) -> (187.7903, 83.4415) construction
  line L2793 (187.7903, 83.4415) -> (187.8212, 83.2764) construction
  line L2794 (187.8212, 83.2764) -> (187.8528, 83.1113) construction
  line L2795 (187.8528, 83.1113) -> (187.8788, 82.9792) construction
  line L2796 (187.8788, 82.9792) -> (187.8986, 82.8801) construction
  line L2797 (187.8986, 82.8801) -> (187.912, 82.814) construction
  line L2798 (187.912, 82.814) -> (187.9188, 82.7809) construction
  spline S37 degree 5 poles (187.9372, 93.9655) (187.9249, 93.9372) (187.9012, 93.8802) (187.868, 93.7938) (187.8281, 93.6771) (187.7842, 93.5289) (187.7447, 93.3792) (187.7079, 93.2286) (187.6725, 93.0774) (187.638, 92.9259) (187.6046, 92.774) (187.5726, 92.6217) (187.5424, 92.4688) (187.5144, 92.3152) (187.4885, 92.1609) (187.4646, 92.006) (187.4423, 91.8506) (187.4215, 91.6948) (187.4019, 91.5386) (187.3835, 91.3821) (187.3662, 91.2253) (187.3502, 91.0682) (187.3355, 90.9107) (187.3222, 90.7529) (187.3102, 90.5947) (187.2995, 90.4362) (187.29, 90.2774) (187.2816, 90.1183) (187.2743, 89.9589) (187.2682, 89.7993) (187.2631, 89.6395) (187.2591, 89.4794) (187.2563, 89.3191) (187.2544, 89.1585) (187.2537, 88.9977) (187.254, 88.8367) (187.2554, 88.6755) (187.2578, 88.5141) (187.2612, 88.3525) (187.2655, 88.1907) (187.2709, 88.0288) (187.2772, 87.8666) (187.2845, 87.7043) (187.2928, 87.5419) (187.302, 87.3793) (187.3121, 87.2165) (187.3232, 87.0536) (187.3353, 86.8905) (187.3482, 86.7273) (187.362, 86.564) (187.3768, 86.4005) (187.3924, 86.2369) (187.409, 86.0732) (187.4264, 85.9094) (187.4447, 85.7455) (187.4639, 85.5815) (187.484, 85.4174) (187.5049, 85.2532) (187.5266, 85.0889) (187.5492, 84.9245) (187.5727, 84.76) (187.597, 84.5954) (187.6222, 84.4308) (187.6481, 84.266) (187.6749, 84.1013) (187.7026, 83.9364) (187.731, 83.7715) (187.7602, 83.6065) (187.7903, 83.4415) (187.8212, 83.2764) (187.8528, 83.1113) (187.8788, 82.9792) (187.8986, 82.8801) (187.912, 82.814) (187.9188, 82.7809) knots 0 0 0 0 0 0 0.01428571 0.02857143 0.04285714 0.05714286 0.07142857 0.08571429 0.1 0.11428571 0.12857143 0.14285714 0.15714286 0.17142857 0.18571429 0.2 0.21428571 0.22857143 0.24285714 0.25714286 0.27142857 0.28571429 0.3 0.31428571 0.32857143 0.34285714 0.35714286 0.37142857 0.38571429 0.4 0.41428571 0.42857143 0.44285714 0.45714286 0.47142857 0.48571429 0.5 0.51428571 0.52857143 0.54285714 0.55714286 0.57142857 0.58571429 0.6 0.61428571 0.62857143 0.64285714 0.65714286 0.67142857 0.68571429 0.7 0.71428571 0.72857143 0.74285714 0.75714286 0.77142857 0.78571429 0.8 0.81428571 0.82857143 0.84285714 0.85714286 0.87142857 0.88571429 0.9 0.91428571 0.92857143 0.94285714 0.95714286 0.97142857 0.98571429 1 1 1 1 1 1
  line L2799 (187.9372, 93.9655) -> (187.9249, 93.9372) construction
  line L2800 (187.9249, 93.9372) -> (187.9012, 93.8802) construction
  line L2801 (187.9012, 93.8802) -> (187.868, 93.7938) construction
  line L2802 (187.868, 93.7938) -> (187.8281, 93.6771) construction
  line L2803 (187.8281, 93.6771) -> (187.7842, 93.5289) construction
  line L2804 (187.7842, 93.5289) -> (187.7447, 93.3792) construction
  line L2805 (187.7447, 93.3792) -> (187.7079, 93.2286) construction
  line L2806 (187.7079, 93.2286) -> (187.6725, 93.0774) construction
  line L2807 (187.6725, 93.0774) -> (187.638, 92.9259) construction
  line L2808 (187.638, 92.9259) -> (187.6046, 92.774) construction
  line L2809 (187.6046, 92.774) -> (187.5726, 92.6217) construction
  line L2810 (187.5726, 92.6217) -> (187.5424, 92.4688) construction
  line L2811 (187.5424, 92.4688) -> (187.5144, 92.3152) construction